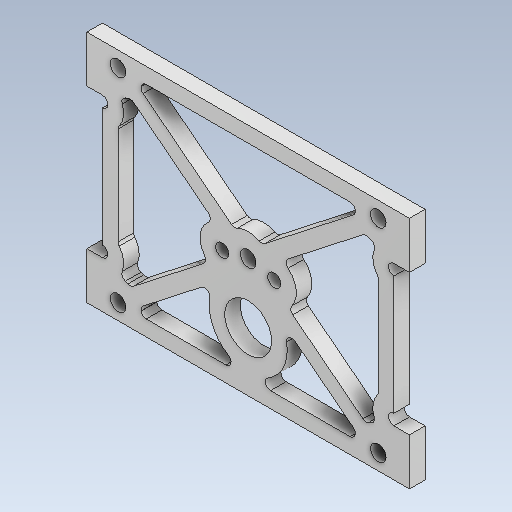
# Autodesk Inventor part: 横回転フレーム改２
Saved by Autodesk Inventor 2020 (Build 240168000, 168)
## iProperties
Created: 2020-02-25
Part Number: 横回転フレーム改２
Material: アルミニウム 2014-T4
Document SubType Name: Modeling
Designer: tanjihayato
Density: 2.8 g/cm^3
Appearance: サテン
Mass: 10.2571 g
Surface Area: 44.4953 cm^2
Volume: 3.66325 cm^3
Author: tanjihayato
Autodesk Inventor part; units mm, degrees
ref_plane "YZ Plane" through (0, 0, 0) normal (1, 0, 0) x (0, 1, 0)
ref_plane "XZ Plane" through (0, 0, 0) normal (0, 1, 0) x (-1, 0, 0)
ref_plane "XY Plane" through (0, 0, 0) normal (0, 0, 1) x (1, 0, 0)
sketch "スケッチ1" plane through (0, 0, 0) normal (0, 0, 1) x (1, 0, 0)
  line L0 (0, 0) -> (0, 4) construction
  line L1 (0, 0) -> (8.6476, -12.2564)
  line L2 (8.6476, -12.2564) -> (-0.2755, 4.5179)
  circle A0 centre (3.0119, -1.6621) radius 4
  line L3 (-57.3278, -140) -> (69.8706, -140)
  line L4 (3.0119, -1.6621) -> (117.7837, 59.3906)
  circle A1 centre (0, 0) radius 23.1
  circle A2 centre (0, -29.1039) radius 6.0039
  line L5 (0, 0) -> (0, -29.1039) construction
  circle A3 centre (0, -29.1039) radius 16.55
  circle A4 centre (0, -7.5039) radius 5.05
  circle A5 centre (0, 4) radius 3
  circle A6 centre (0, -7.5039) radius 20.05
  circle A7 centre (-14, 10.2376) radius 2.55
  circle A8 centre (14, 10.2376) radius 2.55
  circle A9 centre (14, -25.2454) radius 2.55
  circle A10 centre (-14, -25.2454) radius 2.55
  circle A11 centre (-14, 10.2376) radius 14
  circle A12 centre (14, 10.2376) radius 14
  circle A13 centre (14, -25.2454) radius 14
  circle A14 centre (-14, -25.2454) radius 14
  line L6 (-14, 10.2376) -> (-14, -25.2454) construction
  line L7 (-14, -25.2454) -> (14, -25.2454) construction
  circle A15 centre (0, 0) radius 9
  line L8 (-0.2755, 4.5179) -> (3.4816, -2.5449) construction
  line L9 (-2.9462, 3.0973) -> (0.8109, -3.9656)
  line L10 (6.1522, -1.1243) -> (2.3951, 5.9386)
  arc A16 (2.3951, 5.9386) -> (-2.9462, 3.0973) centre (-0.2755, 4.5179) ccw
  arc A17 (0.8109, -3.9656) -> (6.1522, -1.1243) centre (3.4816, -2.5449) ccw
  line L11 (-5, 2.8868) -> (5, 2.8868) construction
  line L12 (5, 2.8868) -> (0, -5.7735) construction
  line L13 (0, -5.7735) -> (-5, 2.8868) construction
  circle A18 centre (-5, 2.8868) radius 1.5
  circle A19 centre (5, 2.8868) radius 1.5
  circle A20 centre (0, -5.7735) radius 1.5
  line L14 (-28, 22.5965) -> (-28, -43.3295)
  line L15 (28, 22.9271) -> (28, -43.0008)
  line L16 (-28, 26.1991) -> (28, 26.1991)
  circle A21 centre (0, 0) radius 25.1
  line L17 (-28, -18.848) -> (28, -18.848)
  circle A22 centre (0, -29.1039) radius 8.0039
  circle A23 centre (-25, 23.1991) radius 3
  circle A24 centre (25, 23.1991) radius 3
  circle A25 centre (25, -38.2069) radius 3
  circle A26 centre (-25, -38.2069) radius 3
  circle A27 centre (-25, -15.848) radius 3
  circle A28 centre (25, -15.848) radius 3
  circle A29 centre (-25, -15.848) radius 4.5
  circle A30 centre (25, -15.848) radius 4.5
  circle A31 centre (0, -7.5039) radius 4.5
  circle A32 centre (0, -29.1039) radius 17.55
  circle A33 centre (0, -7.5039) radius 6.05
  point P0 (1.603, 0.9865)
  dimension "d0" = 4
  dimension "d1" = 15
  dimension "d2" = 18.4133
  dimension "d3" = 19
  dimension "d4" = 8
  dimension "d5" = 12
  dimension "d6" = 140
  dimension "d7" = 130
  dimension "d8" = 46.2
  dimension "d9" = 29.1039
  dimension "d10" = 33.1
  dimension "d11" = 10.1
  dimension "d12" = 6
  dimension "d13" = 40.1
  dimension "d14" = 28
  dimension "d15" = 28
  dimension "d16" = 28
  dimension "d17" = 28
  dimension "d18" = 18
  dimension "d19" = 8
  dimension "d20" = 6.05
  dimension "d21" = 3
  dimension "d22" = 3
  dimension "d23" = 3
  dimension "d24" = 10
  dimension "d25" = 2
  dimension "d26" = 2
  dimension "d27" = 6
  dimension "d28" = 6
  dimension "d29" = 6
  dimension "d30" = 6
  dimension "d31" = 6
  dimension "d32" = 6
  dimension "d33" = 9
  dimension "d34" = 9
  dimension "d35" = 9
  dimension "d36" = 5.1
  dimension "d37" = 1
  dimension "d38" = 1
  dimension "d39" = 56
  dimension "d40" = 28
  constraints: 38 end point, 34 centre point, 26 tangent, 16 coincident, 8 point on line, 5 vertical, 4 point on circle, 3 equal radius, 3 horizontal, 3 perpendicular, 1 midpoint, 1 parallel, 7 other
  measures "d0" distance of L0.start L0.end
  measures "d1" distance of L0.start L1.end
  measures "d2" distance of L0.end L1.end
  measures "d3" distance of L1.end L2.end
  measures "d4" diameter of A0
  measures "d5" distance of L1.end L4.start
  measures "d6" distance from line of L3 L0.start
  measures "d7" distance of L4.start L4.end
  measures "d8" diameter of A1
  measures "d9" distance of L5.end L0.start
  measures "d10" diameter of A3
  measures "d11" diameter of A4
  measures "d12" diameter of A5
  measures "d13" diameter of A6
  measures "d14" diameter of A11
  measures "d15" diameter of A12
  measures "d16" diameter of A13
  measures "d17" diameter of A14
  measures "d18" diameter of A15
  measures "d19" distance of L2.end L8.end
  measures "d20" diameter of A17
  measures "d21" diameter of A18
  measures "d22" diameter of A19
  measures "d23" diameter of A20
  measures "d24" distance of L11.end L12.end
  measures "d25" radial gap between concentric circles of A1 A21
  measures "d26" radial gap between concentric circles of A2 A22
  measures "d27" diameter of A23
  measures "d28" diameter of A24
  measures "d29" diameter of A25
  measures "d30" diameter of A26
  measures "d31" diameter of A27
  measures "d32" diameter of A28
  measures "d33" diameter of A29
  measures "d34" diameter of A30
  measures "d35" diameter of A31
  measures "d36" diameter of A7
  measures "d37" radial gap between concentric circles of A3 A32
  measures "d38" radial gap between concentric circles of A4 A33
  measures "d39" distance between parallel lines of L15 L14
  measures "d40" distance from line of A6.centre L15
sketch "スケッチ2" plane through (0, 0, 0) normal (0, 0, 1) x (1, 0, 0)
  circle A0 centre (25, 23.1991) radius 3 construction
  circle A1 centre (-25, 23.1991) radius 3 construction
  circle A2 centre (-25, -15.848) radius 3 construction
  circle A3 centre (25, -15.848) radius 3 construction
  circle A4 centre (-5, 2.8868) radius 1.5 construction
  circle A5 centre (5, 2.8868) radius 1.5 construction
  circle A6 centre (0, 4) radius 3 construction
  circle A7 centre (0, -7.5039) radius 4.5 projected
  line L0 (-31, 26.1991) -> (31, 26.1991)
  line L1 (31, 26.1991) -> (31, 17.1991)
  line L2 (31, 17.1991) -> (28, 17.1991)
  line L3 (28, 17.1991) -> (28, -9.848)
  line L4 (28, -9.848) -> (31, -9.848)
  line L5 (31, -9.848) -> (31, -18.848)
  line L6 (31, -18.848) -> (-31, -18.848)
  line L7 (-31, -18.848) -> (-31, -9.848)
  line L8 (-31, -9.848) -> (-28, -9.848)
  line L9 (-28, -9.848) -> (-28, 17.1991)
  line L10 (-28, 17.1991) -> (-31, 17.1991)
  line L11 (-31, 17.1991) -> (-31, 26.1991)
  circle A8 centre (-28, 16.1491) radius 1.05
  circle A9 centre (-28, -8.798) radius 1.05
  circle A10 centre (28, -8.798) radius 1.05
  circle A11 centre (28, 16.1491) radius 1.05
  circle A12 centre (-25, 23.1991) radius 1.5
  circle A13 centre (25, 23.1991) radius 1.5
  circle A14 centre (25, -15.848) radius 1.5
  circle A15 centre (-25, -15.848) radius 1.5
  circle A16 centre (0, 4) radius 1.5
  circle A17 centre (-5, 2.8868) radius 1.25
  circle A18 centre (5, 2.8868) radius 1.25
  point P0 (0, 0)
  point P1 (28, -9.848)
  point P2 (28, -7.748)
  point P3 (28, 15.0991)
  point P4 (-28, 15.0991)
  point P5 (-28, -7.748)
  dimension "d41" = 9
  dimension "d42" = 3
  dimension "d43" = 3
  dimension "d44" = 9
  dimension "d46" = 3
  dimension "d47" = 3
  dimension "d48" = 2.1
  dimension "d49" = 2.1
  dimension "d50" = 2.1
  dimension "d51" = 2.1
  dimension "d52" = 3
  dimension "d53" = 3
  dimension "d54" = 3
  dimension "d55" = 3
  dimension "d56" = 3
  dimension "d57" = 2.5
  dimension "d58" = 2.5
  constraints: 24 end point, 11 centre point, 9 point on line, 8 tangent, 7 coincident, 5 perpendicular, 2 horizontal, 1 collinear, 1 vertical
  measures "d41" distance of L0.end L1.end
  measures "d42" distance of L1.end L2.end
  measures "d43" distance of L3.end L4.end
  measures "d44" distance of L4.end L5.end
  measures "d46" distance of L7.end L8.end
  measures "d47" distance of L9.end L10.end
  measures "d48" diameter of A8
  measures "d49" diameter of A9
  measures "d50" diameter of A10
  measures "d51" diameter of A11
  measures "d52" diameter of A12
  measures "d53" diameter of A13
  measures "d54" diameter of A14
  measures "d55" diameter of A15
  measures "d56" diameter of A16
  measures "d57" diameter of A17
  measures "d58" diameter of A18
extrude "押し出し1" add sketch "スケッチ2" along normal blind 3 contours L0 L1 L2 A11 L3 A10 L4 L5 L6 L7 L8 A9 L9 A8 L10 L11
sketch "スケッチ3" plane through (0, 0, 3) normal (0, 0, 1) x (1, 0, 0)
  arc A0 (-28, 15.0991) -> (-28, 17.1991) centre (-28, 16.1491) ccw projected
  line L0 (-28, 15.0991) -> (-28, -7.748) projected
  arc A1 (-28, -9.848) -> (-28, -7.748) centre (-28, -8.798) ccw projected
  line L1 (-28, -9.848) -> (-31, -9.848) projected
  line L2 (-31, -9.848) -> (-31, -18.848) projected
  line L3 (-31, -18.848) -> (31, -18.848) projected
  line L4 (31, -18.848) -> (31, -9.848) projected
  line L5 (31, -9.848) -> (28, -9.848) projected
  arc A2 (28, -7.748) -> (28, -9.848) centre (28, -8.798) ccw projected
  line L6 (28, -7.748) -> (28, 15.0991) projected
  arc A3 (28, 17.1991) -> (28, 15.0991) centre (28, 16.1491) ccw projected
  line L7 (28, 17.1991) -> (31, 17.1991) projected
  line L8 (31, 17.1991) -> (31, 26.1991) projected
  line L9 (31, 26.1991) -> (-31, 26.1991) projected
  line L10 (-31, 26.1991) -> (-31, 17.1991) projected
  line L11 (-31, 17.1991) -> (-28, 17.1991) projected
  circle A4 centre (5, 2.8868) radius 1.25 projected
  circle A5 centre (0, 4) radius 1.5 projected
  circle A6 centre (-25, -15.848) radius 1.5 projected
  circle A7 centre (25, -15.848) radius 1.5 projected
  circle A8 centre (25, 23.1991) radius 1.5 projected
  circle A9 centre (-25, 23.1991) radius 1.5 projected
  circle A10 centre (0, -7.5039) radius 4.5 projected
  circle A11 centre (-5, 2.8868) radius 1.25 projected
  line L12 (-28, 23.1991) -> (28, 23.1991)
  line L13 (28, 23.1991) -> (28, 20.1991)
  arc A12 (28, 20.1991) -> (25, 13.4283) centre (28, 16.1491) ccw
  line L14 (25, 13.4283) -> (25, -6.0773)
  arc A13 (25, -6.0773) -> (28, -12.848) centre (28, -8.798) ccw
  line L15 (28, -12.848) -> (28, -15.848)
  line L16 (28, -15.848) -> (-28, -15.848)
  line L17 (-28, -15.848) -> (-28, -12.848)
  arc A14 (-28, -12.848) -> (-25, -6.0773) centre (-28, -8.798) ccw
  line L18 (-25, -6.0773) -> (-25, 13.4283)
  arc A15 (-25, 13.4283) -> (-28, 20.1991) centre (-28, 16.1491) ccw
  line L19 (-28, 20.1991) -> (-28, 23.1991)
  circle A16 centre (-25, 23.1991) radius 4.5
  circle A17 centre (25, 23.1991) radius 4.5
  circle A18 centre (25, -15.848) radius 4.5
  circle A19 centre (-25, -15.848) radius 4.5
  circle A20 centre (0, -7.5039) radius 7.5
  circle A21 centre (-5, 2.8868) radius 4.25
  circle A22 centre (0, 4) radius 4.5
  circle A23 centre (5, 2.8868) radius 4.25
  line L20 (-25, 23.1991) -> (25, -15.848) construction
  line L21 (-25.9232, 22.0168) -> (24.0768, -17.0302)
  line L22 (25.9232, -14.6658) -> (-24.0768, 24.3813)
  arc A24 (-24.0768, 24.3813) -> (-25.9232, 22.0168) centre (-25, 23.1991) ccw
  arc A25 (24.0768, -17.0302) -> (25.9232, -14.6658) centre (25, -15.848) ccw
  line L23 (25, 23.1991) -> (-25, -15.848) construction
  line L24 (24.0768, 24.3813) -> (-25.9232, -14.6658)
  line L25 (-24.0768, -17.0302) -> (25.9232, 22.0168)
  arc A26 (25.9232, 22.0168) -> (24.0768, 24.3813) centre (25, 23.1991) ccw
  arc A27 (-25.9232, -14.6658) -> (-24.0768, -17.0302) centre (-25, -15.848) ccw
  arc A28 (3.776, -13.984) -> (4.2795, -15.848) centre (4.2795, -14.848) ccw
  arc A29 (-4.2795, -15.848) -> (-3.776, -13.984) centre (-4.2795, -14.848) ccw
  point P0 (0, 0)
  point P1 (0, 3.6755)
  point P2 (0, 3.6755)
  point P3 (-5.8186, -2.7717)
  point P4 (-20.733, -14.4189)
  point P5 (-20.5, -15.848)
  point P6 (20.5, -15.848)
  point P7 (20.733, -14.4189)
  point P8 (5.8186, -2.7717)
  point P9 (24.8555, 18.7014)
  point P10 (22.5794, 19.4055)
  point P11 (6.5128, 6.8584)
  point P12 (7.6755, -0.4154)
  point P13 (22.5794, -12.0545)
  point P14 (24.8555, -11.3504)
  point P15 (2.6425, 7.6424)
  point P16 (20.733, 21.77)
  point P17 (20.5, 23.1991)
  point P18 (-20.5, 23.1991)
  point P19 (-20.733, 21.77)
  point P20 (-2.6425, 7.6424)
  point P21 (-24.8555, -11.3504)
  point P22 (-22.5794, -12.0545)
  point P23 (-7.6755, -0.4154)
  point P24 (-6.5128, 6.8584)
  point P25 (-22.5794, 19.4055)
  point P26 (-24.8555, 18.7014)
  dimension "d61" = 3
  dimension "d62" = 3
  dimension "d63" = 3
  dimension "d64" = 3
  dimension "d65" = 3
  dimension "d66" = 3
  dimension "d67" = 3
  dimension "d68" = 3
  dimension "d69" = 3
  dimension "d70" = 3
  dimension "d71" = 3
  dimension "d72" = 2
  dimension "d73" = 2
  constraints: 32 end point, 22 point on circle, 18 centre point, 12 tangent, 2 concentric, 2 midpoint, 2 parallel, 2 point on line, 11 other
  measures "d61" distance between parallel lines of L9 L12
  measures "d62" radial gap between concentric circles of A9 A16
  measures "d63" radial gap between concentric circles of A8 A17
  measures "d64" radial gap between concentric circles of A7 A18
  measures "d65" radial gap between concentric circles of A6 A19
  measures "d66" radial gap between concentric circles of A10 A20
  measures "d67" radial gap between concentric circles of A11 A21
  measures "d68" radial gap between concentric circles of A5 A22
  measures "d69" radial gap between concentric circles of A4 A23
  measures "d70" diameter of A25
  measures "d71" diameter of A27
  measures "d72" diameter of A28
  measures "d73" diameter of A29
extrude "押し出し2" cut sketch "スケッチ3" against normal blind 10 contours A16 L21 A21 L24 A19 A14 L18 A15 | L12 A17 L24 A22 L22 A16 | A19 L25 A20 A29 L16 | L16 A28 A20 L21 A18 | A12 L14 A13 A18 L22 A23 L25 A17
fillet "フィレット1" radius 1 28 edges at (-5.8186, -2.7717, 1.5) (-20.733, -14.4189, 1.5) (-20.5, -15.848, 1.5) (-25, -6.0773, 1.5) (-25, 13.4283, 1.5) (-24.8555, -11.3504, 1.5) (-22.5794, -12.0545, 1.5) (-7.6755, -0.4154, 1.5) (-6.5128, 6.8584, 1.5) (-22.5794, 19.4055, 1.5) (-24.8555, 18.7014, 1.5) (20.5, -15.848, 1.5) (20.733, -14.4189, 1.5) (5.8186, -2.7717, 1.5) (20.733, 21.77, 1.5) (2.6425, 7.6424, 1.5) (20.5, 23.1991, 1.5) (-20.5, 23.1991, 1.5) (-20.733, 21.77, 1.5) (-2.6425, 7.6424, 1.5) (25, 13.4283, 1.5) (25, -6.0773, 1.5) (24.8555, 18.7014, 1.5) (22.5794, 19.4055, 1.5) (6.5128, 6.8584, 1.5) (7.6755, -0.4154, 1.5) (22.5794, -12.0545, 1.5) (24.8555, -11.3504, 1.5)
equation "\"d14\" = d15"
equation "\"d16\" = d15"
equation "\"d17\" = d14"
equation "\"d40\" = 0.5 * d39"
